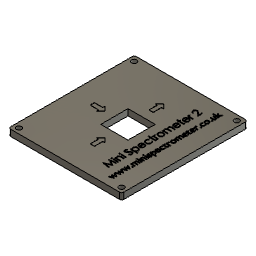
Mini Spectrometer Lid (Autodesk Fusion 360 design; units mm, degrees)
Autodesk Fusion 360 part; units mm, degrees
note: some values were not read from the file. Set by a fixed rule: which sketch regions a step uses.
(part 1 of 2)
sketch "Sketch1" plane through (0, 0, 0) normal (0, 1, 0) x (1, 0, 0)
  line L0 (-27, -30) -> (27, 30) construction
  line L1 (27, 30) -> (27, -30)
  line L2 (27, -30) -> (-27, -30)
  line L3 (-27, 30) -> (27, 30)
  line L4 (-27, -30) -> (-27, 30)
  line L5 (27, -30) -> (-27, 30) construction
  dimension "d1" = 54
  dimension "d2" = 60
  dimension "d3" = 27
  dimension "d29" = 30
  constraint horizontal L2
  constraint perpendicular L2 L4
  constraint parallel L2 L3
  constraint parallel L1 L4
  constraint coincident origin L5
  constraint coincident origin L0
  measures "d1" distance of L3.start L0.end
  measures "d2" distance of L3.start L0.start
  measures "d3" distance of origin L4
  measures "d29" distance of origin L3
extrude "Extrude1" add sketch "Sketch1" along normal blind 3
fillet "Fillet1" radius 1 4 edges at (27, 1.5, 30) (-27, 1.5, 30) (-27, 1.5, -30) (27, 1.5, -30)
sketch "Sketch3" plane through (0, 3, 0) normal (0, 1, 0) x (-1, 0, 0)
  arc A0 (-27, -29) -> (-26, -30) centre (-26, -29) ccw
  line L0 (-26, -30) -> (26, -30)
  arc A1 (26, -30) -> (27, -29) centre (26, -29) ccw
  line L1 (27, -29) -> (27, 29)
  arc A2 (27, 29) -> (26, 30) centre (26, 29) ccw
  line L2 (26, 30) -> (-26, 30)
  arc A3 (-26, 30) -> (-27, 29) centre (-26, 29) ccw
  line L3 (-27, 29) -> (-27, -29)
  circle A4 centre (24.5, -27.5) radius 1.25
  circle A5 centre (-24.5, -27.5) radius 1.25
  circle A6 centre (-24.5, 27.5) radius 1.25
  circle A7 centre (24.5, 27.5) radius 1.25
  line L4 (-6.5, -6.5) -> (-6.5, 6.5)
  line L5 (-6.5, 6.5) -> (6.5, 6.5)
  line L6 (6.5, 6.5) -> (6.5, -6.5)
  line L7 (6.5, -6.5) -> (-6.5, -6.5)
  dimension "d21" = 2.5
  dimension "d22" = 2.5
  dimension "d23" = 2.5
  dimension "d24" = 2.5
  dimension "d25" = 13
  dimension "d26" = 13
  dimension "d30" = 2.5
  dimension "d31" = 2.5
  dimension "d32" = 2.5
  dimension "d33" = 2.5
  dimension "d34" = 2.5
  dimension "d35" = 2.5
  dimension "d36" = 2.5
  dimension "d37" = 2.5
  dimension "d38" = 20.5
  dimension "d39" = 23.5
  constraint horizontal L5
  constraint perpendicular L5 L6
  constraint parallel L5 L7
  constraint parallel L4 L6
  measures "d21" diameter of A4
  measures "d22" diameter of A5
  measures "d23" diameter of A6
  measures "d24" diameter of A7
  measures "d25" distance of L4.start L6.end
  measures "d26" distance of L6.end L5.end
  measures "d30" distance of L2 A7.centre
  measures "d31" distance of L1 A7.centre
  measures "d32" distance of L2 A6.centre
  measures "d33" distance of L3 A6.centre
  measures "d34" distance of L0 A5.centre
  measures "d35" distance of L3 A5.centre
  measures "d36" distance of L0 A4.centre
  measures "d37" distance of L1 A4.centre
  measures "d38" distance of L1 L6
  measures "d39" distance of L0 L7
extrude "Extrude2" cut sketch "Sketch3" against normal blind 3 contours A4 | A5 | A6 | A7 | L4 L5 L6 L7
sketch "Sketch4" plane through (0, 3, 0) normal (0, 1, 0) x (-1, 0, 0)
  line L0 (-6.5, 6.5) -> (6.5, 6.5)
  line L1 (6.5, 6.5) -> (6.5, -6.5)
  line L2 (6.5, -6.5) -> (-6.5, -6.5)
  line L3 (-6.5, -6.5) -> (-6.5, 6.5)
  circle A0 centre (24.5, 27.5) radius 1.25
  circle A1 centre (-24.5, -27.5) radius 1.25
  circle A2 centre (24.5, -27.5) radius 1.25
  circle A3 centre (-24.5, 27.5) radius 1.25
  arc A4 (-27, -29) -> (-26, -30) centre (-26, -29) ccw
  line L4 (-26, -30) -> (26, -30)
  arc A5 (26, -30) -> (27, -29) centre (26, -29) ccw
  line L5 (27, -29) -> (27, 29)
  arc A6 (27, 29) -> (26, 30) centre (26, 29) ccw
  line L6 (26, 30) -> (-26, 30)
  arc A7 (-26, 30) -> (-27, 29) centre (-26, 29) ccw
  line L7 (-27, 29) -> (-27, -29)
  line L8 (11, 0) -> (13, -2)
  line L9 (13, -2) -> (13, -1)
  line L10 (13, -1) -> (17, -1)
  line L11 (17, -1) -> (17, 1)
  line L12 (17, 1) -> (13, 1)
  line L13 (13, 1) -> (13, 2)
  line L14 (13, 2) -> (11, 0)
  line L15 (13, -1) -> (17, -1)
  line L16 (13, -2) -> (13, -1)
  line L17 (11, 0) -> (13, -2)
  line L18 (13, 1) -> (13, 2)
  line L19 (17, 1) -> (13, 1)
  line L20 (17, -1) -> (17, 1)
  line L21 (13, 2) -> (11, 0)
  line L22 (1, 13) -> (1, 17)
  line L23 (2, 13) -> (1, 13)
  line L24 (0, 11) -> (2, 13)
  line L25 (-1, 13) -> (-2, 13)
  line L26 (-1, 17) -> (-1, 13)
  line L27 (1, 17) -> (-1, 17)
  line L28 (-2, 13) -> (0, 11)
  line L29 (1, -15) -> (1, -11)
  line L30 (2, -15) -> (1, -15)
  line L31 (0, -17) -> (2, -15)
  line L32 (-1, -15) -> (-2, -15)
  line L33 (-1, -11) -> (-1, -15)
  line L34 (1, -11) -> (-1, -11)
  line L35 (-2, -15) -> (0, -17)
  constraint perpendicular L2 L9
  constraint perpendicular L9 L10
  constraint perpendicular L10 L11
  constraint perpendicular L11 L12
  constraint perpendicular L12 L13
  constraint perpendicular L8 L14
  constraint perpendicular L15 L16
  constraint perpendicular L15 L20
  constraint perpendicular L19 L20
  constraint perpendicular L18 L19
  constraint perpendicular L17 L21
  constraint perpendicular L22 L23
  constraint perpendicular L22 L27
  constraint perpendicular L26 L27
  constraint perpendicular L25 L26
  constraint perpendicular L24 L28
  constraint perpendicular L29 L30
  constraint perpendicular L29 L34
  constraint perpendicular L33 L34
  constraint perpendicular L32 L33
  constraint perpendicular L31 L35
extrude "Extrude3" cut sketch "Sketch4" against normal blind 0.1 contours L8 L9 L10 L11 L12 L13 L14 L15 L16 L17 L18 L19 L20 L21 | L22 L23 L24 L25 L26 L27 L28 | L29 L30 L31 L32 L33 L34 L35
sketch "Sketch5" plane through (0, 3, 0) normal (0, 1, 0) x (-1, 0, 0)
  line L0 (2, -15) -> (0, -17)
  line L1 (0, -17) -> (-2, -15)
  line L2 (-2, -15) -> (-1, -15)
  line L3 (-1, -15) -> (-1, -11)
  line L4 (-1, -11) -> (1, -11)
  line L5 (1, -11) -> (1, -15)
  line L6 (1, -15) -> (2, -15)
  line L7 (2, 13) -> (0, 11)
  line L8 (0, 11) -> (-2, 13)
  line L9 (-2, 13) -> (-1, 13)
  line L10 (-1, 13) -> (-1, 17)
  line L11 (-1, 17) -> (1, 17)
  line L12 (1, 17) -> (1, 13)
  line L13 (1, 13) -> (2, 13)
  line L14 (13, -2) -> (11, 0)
  line L15 (11, 0) -> (13, 2)
  line L16 (13, 2) -> (13, 1)
  line L17 (13, 1) -> (17, 1)
  line L18 (17, 1) -> (17, -1)
  line L19 (17, -1) -> (13, -1)
  line L20 (13, -1) -> (13, -2)
  line L21 (-6.5, 6.5) -> (6.5, 6.5)
  line L22 (6.5, 6.5) -> (6.5, -6.5)
  line L23 (6.5, -6.5) -> (-6.5, -6.5)
  line L24 (-6.5, -6.5) -> (-6.5, 6.5)
  circle A0 centre (24.5, 27.5) radius 1.25
  circle A1 centre (-24.5, -27.5) radius 1.25
  circle A2 centre (24.5, -27.5) radius 1.25
  circle A3 centre (-24.5, 27.5) radius 1.25
  arc A4 (-27, -29) -> (-26, -30) centre (-26, -29) ccw
  line L25 (-26, -30) -> (26, -30)
  arc A5 (26, -30) -> (27, -29) centre (26, -29) ccw
  line L26 (27, -29) -> (27, 29)
  arc A6 (27, 29) -> (26, 30) centre (26, 29) ccw
  line L27 (26, 30) -> (-26, 30)
  arc A7 (-26, 30) -> (-27, 29) centre (-26, 29) ccw
  line L28 (-27, 29) -> (-27, -29)
  line L29 (-13.2189, 22.3541) -> (-9.8548, 21.8762)
  line L30 (-9.8548, 21.8762) -> (-9.8548, 21.8246)
  line L31 (-9.8548, 21.8246) -> (-12.6145, 20.4565)
  line L32 (-12.6145, 20.4565) -> (-9.8548, 19.0977)
  line L33 (-9.8548, 19.0977) -> (-9.8548, 19.0462)
  line L34 (-9.8548, 19.0462) -> (-13.2189, 18.5636)
  line L35 (-13.2189, 18.5636) -> (-13.2189, 18.8963)
  line L36 (-13.2189, 18.8963) -> (-10.8106, 19.2242)
  line L37 (-10.8106, 19.2242) -> (-13.2189, 20.4143)
  line L38 (-13.2189, 20.4143) -> (-13.2189, 20.4987)
  line L39 (-13.2189, 20.4987) -> (-10.7918, 21.7028)
  line L40 (-10.7918, 21.7028) -> (-13.2189, 22.0308)
  line L41 (-13.2189, 22.0308) -> (-13.2189, 22.3541)
  spline S0 degree 2 poles (-10.0375, 18.0997) (-9.9297, 18.0997) (-9.8501, 18.0248) knots 0 0 0 1 1 1
  spline S1 degree 2 poles (-9.8501, 18.0248) (-9.7704, 17.9451) (-9.7704, 17.8373) knots 0 0 0 1 1 1
  spline S2 degree 2 poles (-9.7704, 17.8373) (-9.7704, 17.7249) (-9.8501, 17.6499) knots 0 0 0 1 1 1
  spline S3 degree 2 poles (-9.8501, 17.6499) (-9.925, 17.5703) (-10.0375, 17.5703) knots 0 0 0 1 1 1
  spline S4 degree 2 poles (-10.0375, 17.5703) (-10.1452, 17.5703) (-10.2249, 17.6499) knots 0 0 0 1 1 1
  spline S5 degree 2 poles (-10.2249, 17.6499) (-10.2999, 17.7249) (-10.2999, 17.8373) knots 0 0 0 1 1 1
  spline S6 degree 2 poles (-10.2999, 17.8373) (-10.2999, 17.9451) (-10.2202, 18.0248) knots 0 0 0 1 1 1
  spline S7 degree 2 poles (-10.2202, 18.0248) (-10.1406, 18.0997) (-10.0375, 18.0997) knots 0 0 0 1 1 1
  line L42 (-10.7309, 17.9967) -> (-10.7309, 17.6734)
  line L43 (-10.7309, 17.6734) -> (-13.2189, 17.6734)
  line L44 (-13.2189, 17.6734) -> (-13.2189, 17.9967)
  line L45 (-13.2189, 17.9967) -> (-10.7309, 17.9967)
  line L46 (-10.7309, 17.0127) -> (-10.7309, 16.6894)
  line L47 (-10.7309, 16.6894) -> (-11.176, 16.6894)
  spline S8 degree 2 poles (-11.176, 16.6894) (-10.6653, 16.3052) (-10.6653, 15.757) knots 0 0 0 1 1 1
  spline S9 degree 2 poles (-10.6653, 15.757) (-10.6653, 15.4759) (-10.8199, 15.251) knots 0 0 0 1 1 1
  spline S10 degree 2 poles (-10.8199, 15.251) (-10.9699, 15.0261) (-11.2182, 14.9324) knots 0 0 0 1 1 1
  spline S11 degree 2 poles (-11.2182, 14.9324) (-11.4618, 14.8387) (-11.9398, 14.8387) knots 0 0 0 1 1 1
  line L48 (-11.9398, 14.8387) -> (-13.2189, 14.8387)
  line L49 (-13.2189, 14.8387) -> (-13.2189, 15.1573)
  line L50 (-13.2189, 15.1573) -> (-12.0335, 15.1573)
  spline S12 degree 2 poles (-12.0335, 15.1573) (-11.5977, 15.1573) (-11.4431, 15.1995) knots 0 0 0 1 1 1
  spline S13 degree 2 poles (-11.4431, 15.1995) (-11.2885, 15.2369) (-11.1807, 15.3213) knots 0 0 0 1 1 1
  spline S14 degree 2 poles (-11.1807, 15.3213) (-11.073, 15.4009) (-11.0167, 15.5274) knots 0 0 0 1 1 1
  spline S15 degree 2 poles (-11.0167, 15.5274) (-10.9605, 15.6539) (-10.9605, 15.8367) knots 0 0 0 1 1 1
  spline S16 degree 2 poles (-10.9605, 15.8367) (-10.9605, 16.0147) (-11.0495, 16.1881) knots 0 0 0 1 1 1
  spline S17 degree 2 poles (-11.0495, 16.1881) (-11.1386, 16.3614) (-11.2979, 16.4833) knots 0 0 0 1 1 1
  spline S18 degree 2 poles (-11.2979, 16.4833) (-11.4572, 16.6051) (-11.6258, 16.6473) knots 0 0 0 1 1 1
  spline S19 degree 2 poles (-11.6258, 16.6473) (-11.7945, 16.6894) (-12.3052, 16.6894) knots 0 0 0 1 1 1
  line L51 (-12.3052, 16.6894) -> (-13.2189, 16.6894)
  line L52 (-13.2189, 16.6894) -> (-13.2189, 17.0127)
  line L53 (-13.2189, 17.0127) -> (-10.7309, 17.0127)
  spline S20 degree 2 poles (-10.0375, 14.3046) (-9.9297, 14.3046) (-9.8501, 14.2296) knots 0 0 0 1 1 1
  spline S21 degree 2 poles (-9.8501, 14.2296) (-9.7704, 14.1499) (-9.7704, 14.0422) knots 0 0 0 1 1 1
  spline S22 degree 2 poles (-9.7704, 14.0422) (-9.7704, 13.9297) (-9.8501, 13.8548) knots 0 0 0 1 1 1
  spline S23 degree 2 poles (-9.8501, 13.8548) (-9.925, 13.7751) (-10.0375, 13.7751) knots 0 0 0 1 1 1
  spline S24 degree 2 poles (-10.0375, 13.7751) (-10.1452, 13.7751) (-10.2249, 13.8548) knots 0 0 0 1 1 1
  spline S25 degree 2 poles (-10.2249, 13.8548) (-10.2999, 13.9297) (-10.2999, 14.0422) knots 0 0 0 1 1 1
  spline S26 degree 2 poles (-10.2999, 14.0422) (-10.2999, 14.1499) (-10.2202, 14.2296) knots 0 0 0 1 1 1
  spline S27 degree 2 poles (-10.2202, 14.2296) (-10.1406, 14.3046) (-10.0375, 14.3046) knots 0 0 0 1 1 1
  line L54 (-10.7309, 14.2015) -> (-10.7309, 13.8782)
  line L55 (-10.7309, 13.8782) -> (-13.2189, 13.8782)
  line L56 (-13.2189, 13.8782) -> (-13.2189, 14.2015)
  line L57 (-13.2189, 14.2015) -> (-10.7309, 14.2015)
  line L58 (-12.591, 12.3414) -> (-12.4224, 12.0556)
  spline S28 degree 2 poles (-12.4224, 12.0556) (-12.9752, 11.7557) (-12.9752, 11.3574) knots 0 0 0 1 1 1
  spline S29 degree 2 poles (-12.9752, 11.3574) (-12.9752, 11.0997) (-12.8112, 10.917) knots 0 0 0 1 1 1
  spline S30 degree 2 poles (-12.8112, 10.917) (-12.6473, 10.7343) (-12.4036, 10.7343) knots 0 0 0 1 1 1
  spline S31 degree 2 poles (-12.4036, 10.7343) (-12.2115, 10.7343) (-12.0147, 10.8889) knots 0 0 0 1 1 1
  spline S32 degree 2 poles (-12.0147, 10.8889) (-11.8179, 11.0435) (-11.5509, 11.4043) knots 0 0 0 1 1 1
  spline S33 degree 2 poles (-11.5509, 11.4043) (-11.2791, 11.7604) (-11.1479, 11.8869) knots 0 0 0 1 1 1
  spline S34 degree 2 poles (-11.1479, 11.8869) (-11.012, 12.0087) (-10.8621, 12.0696) knots 0 0 0 1 1 1
  spline S35 degree 2 poles (-10.8621, 12.0696) (-10.7075, 12.1258) (-10.5529, 12.1258) knots 0 0 0 1 1 1
  spline S36 degree 2 poles (-10.5529, 12.1258) (-10.2249, 12.1258) (-10, 11.8963) knots 0 0 0 1 1 1
  spline S37 degree 2 poles (-10, 11.8963) (-9.7704, 11.662) (-9.7704, 11.3106) knots 0 0 0 1 1 1
  spline S38 degree 2 poles (-9.7704, 11.3106) (-9.7704, 11.0341) (-9.911, 10.828) knots 0 0 0 1 1 1
  spline S39 degree 2 poles (-9.911, 10.828) (-10.0469, 10.6218) (-10.3186, 10.4297) knots 0 0 0 1 1 1
  line L59 (-10.3186, 10.4297) -> (-10.5295, 10.7015)
  spline S40 degree 2 poles (-10.5295, 10.7015) (-10.3514, 10.8327) (-10.2343, 10.9732) knots 0 0 0 1 1 1
  spline S41 degree 2 poles (-10.2343, 10.9732) (-10.1171, 11.1138) (-10.1171, 11.3199) knots 0 0 0 1 1 1
  spline S42 degree 2 poles (-10.1171, 11.3199) (-10.1171, 11.5214) (-10.239, 11.6526) knots 0 0 0 1 1 1
  spline S43 degree 2 poles (-10.239, 11.6526) (-10.3608, 11.7791) (-10.5482, 11.7791) knots 0 0 0 1 1 1
  spline S44 degree 2 poles (-10.5482, 11.7791) (-10.7356, 11.7791) (-10.8762, 11.6667) knots 0 0 0 1 1 1
  spline S45 degree 2 poles (-10.8762, 11.6667) (-11.012, 11.5495) (-11.3119, 11.1466) knots 0 0 0 1 1 1
  spline S46 degree 2 poles (-11.3119, 11.1466) (-11.6118, 10.739) (-11.8648, 10.5562) knots 0 0 0 1 1 1
  spline S47 degree 2 poles (-11.8648, 10.5562) (-12.1178, 10.3688) (-12.3989, 10.3688) knots 0 0 0 1 1 1
  spline S48 degree 2 poles (-12.3989, 10.3688) (-12.7644, 10.3688) (-13.0361, 10.6546) knots 0 0 0 1 1 1
  spline S49 degree 2 poles (-13.0361, 10.6546) (-13.3032, 10.9357) (-13.3032, 11.3106) knots 0 0 0 1 1 1
  spline S50 degree 2 poles (-13.3032, 11.3106) (-13.3032, 11.9712) (-12.591, 12.3414) knots 0 0 0 1 1 1
  line L60 (-10.7309, 9.7082) -> (-10.7309, 9.3896)
  line L61 (-10.7309, 9.3896) -> (-11.1854, 9.3896)
  spline S51 degree 2 poles (-11.1854, 9.3896) (-10.6653, 9.01) (-10.6653, 8.4009) knots 0 0 0 1 1 1
  spline S52 degree 2 poles (-10.6653, 8.4009) (-10.6653, 7.8762) (-11.0542, 7.4967) knots 0 0 0 1 1 1
  spline S53 degree 2 poles (-11.0542, 7.4967) (-11.4384, 7.1171) (-11.9819, 7.1171) knots 0 0 0 1 1 1
  spline S54 degree 2 poles (-11.9819, 7.1171) (-12.5254, 7.1171) (-12.9143, 7.492) knots 0 0 0 1 1 1
  spline S55 degree 2 poles (-12.9143, 7.492) (-13.3032, 7.8668) (-13.3032, 8.3916) knots 0 0 0 1 1 1
  spline S56 degree 2 poles (-13.3032, 8.3916) (-13.3032, 8.9632) (-12.7925, 9.3896) knots 0 0 0 1 1 1
  line L62 (-12.7925, 9.3896) -> (-14.1278, 9.3896)
  line L63 (-14.1278, 9.3896) -> (-14.1278, 9.7082)
  line L64 (-14.1278, 9.7082) -> (-10.7309, 9.7082)
  spline S57 degree 2 poles (-11.9866, 7.4357) (-11.5696, 7.4357) (-11.2744, 7.7262) knots 0 0 0 1 1 1
  spline S58 degree 2 poles (-11.2744, 7.7262) (-10.9746, 8.012) (-10.9746, 8.429) knots 0 0 0 1 1 1
  spline S59 degree 2 poles (-10.9746, 8.429) (-10.9746, 8.846) (-11.2697, 9.1319) knots 0 0 0 1 1 1
  spline S60 degree 2 poles (-11.2697, 9.1319) (-11.5602, 9.413) (-11.9913, 9.413) knots 0 0 0 1 1 1
  spline S61 degree 2 poles (-11.9913, 9.413) (-12.4224, 9.413) (-12.7175, 9.1225) knots 0 0 0 1 1 1
  spline S62 degree 2 poles (-12.7175, 9.1225) (-13.008, 8.832) (-13.008, 8.429) knots 0 0 0 1 1 1
  spline S63 degree 2 poles (-13.008, 8.429) (-13.008, 8.0214) (-12.7129, 7.7309) knots 0 0 0 1 1 1
  spline S64 degree 2 poles (-12.7129, 7.7309) (-12.413, 7.4357) (-11.9866, 7.4357) knots 0 0 0 1 1 1
  line L65 (-12.413, 4.423) -> (-12.5535, 4.1513)
  spline S65 degree 2 poles (-12.5535, 4.1513) (-13.3032, 4.5542) (-13.3032, 5.3414) knots 0 0 0 1 1 1
  spline S66 degree 2 poles (-13.3032, 5.3414) (-13.3032, 5.9036) (-12.919, 6.2691) knots 0 0 0 1 1 1
  spline S67 degree 2 poles (-12.919, 6.2691) (-12.5301, 6.6345) (-11.9866, 6.6345) knots 0 0 0 1 1 1
  spline S68 degree 2 poles (-11.9866, 6.6345) (-11.4431, 6.6345) (-11.0542, 6.2691) knots 0 0 0 1 1 1
  spline S69 degree 2 poles (-11.0542, 6.2691) (-10.6653, 5.8989) (-10.6653, 5.3601) knots 0 0 0 1 1 1
  spline S70 degree 2 poles (-10.6653, 5.3601) (-10.6653, 4.8166) (-11.0261, 4.4511) knots 0 0 0 1 1 1
  spline S71 degree 2 poles (-11.0261, 4.4511) (-11.3869, 4.081) (-12.01, 4.0669) knots 0 0 0 1 1 1
  line L66 (-12.01, 4.0669) -> (-12.01, 6.3066)
  spline S72 degree 2 poles (-12.01, 6.3066) (-12.4598, 6.2925) (-12.7363, 6.0254) knots 0 0 0 1 1 1
  spline S73 degree 2 poles (-12.7363, 6.0254) (-13.008, 5.7537) (-13.008, 5.3695) knots 0 0 0 1 1 1
  spline S74 degree 2 poles (-13.008, 5.3695) (-13.008, 4.7369) (-12.413, 4.423) knots 0 0 0 1 1 1
  spline S75 degree 2 poles (-11.7336, 4.423) (-11.3775, 4.4886) (-11.176, 4.751) knots 0 0 0 1 1 1
  spline S76 degree 2 poles (-11.176, 4.751) (-10.9746, 5.0134) (-10.9746, 5.3554) knots 0 0 0 1 1 1
  spline S77 degree 2 poles (-10.9746, 5.3554) (-10.9746, 6.0582) (-11.7336, 6.2738) knots 0 0 0 1 1 1
  line L67 (-11.7336, 6.2738) -> (-11.7336, 4.423)
  line L68 (-11.2463, 1.0402) -> (-11.4056, 1.2932)
  spline S78 degree 2 poles (-11.4056, 1.2932) (-10.9699, 1.6212) (-10.9699, 2.1928) knots 0 0 0 1 1 1
  spline S79 degree 2 poles (-10.9699, 2.1928) (-10.9699, 2.6426) (-11.2604, 2.9471) knots 0 0 0 1 1 1
  spline S80 degree 2 poles (-11.2604, 2.9471) (-11.5462, 3.2517) (-11.9726, 3.2517) knots 0 0 0 1 1 1
  spline S81 degree 2 poles (-11.9726, 3.2517) (-12.3989, 3.2517) (-12.7035, 2.9518) knots 0 0 0 1 1 1
  spline S82 degree 2 poles (-12.7035, 2.9518) (-13.008, 2.6519) (-13.008, 2.1928) knots 0 0 0 1 1 1
  spline S83 degree 2 poles (-13.008, 2.1928) (-13.008, 1.6446) (-12.5723, 1.2932) knots 0 0 0 1 1 1
  line L69 (-12.5723, 1.2932) -> (-12.741, 1.0402)
  spline S84 degree 2 poles (-12.741, 1.0402) (-13.0127, 1.2276) (-13.158, 1.5462) knots 0 0 0 1 1 1
  spline S85 degree 2 poles (-13.158, 1.5462) (-13.3032, 1.8601) (-13.3032, 2.2256) knots 0 0 0 1 1 1
  spline S86 degree 2 poles (-13.3032, 2.2256) (-13.3032, 2.8019) (-12.9237, 3.1908) knots 0 0 0 1 1 1
  spline S87 degree 2 poles (-12.9237, 3.1908) (-12.5442, 3.575) (-11.996, 3.575) knots 0 0 0 1 1 1
  spline S88 degree 2 poles (-11.996, 3.575) (-11.4478, 3.575) (-11.0589, 3.1861) knots 0 0 0 1 1 1
  spline S89 degree 2 poles (-11.0589, 3.1861) (-10.6653, 2.7925) (-10.6653, 2.1787) knots 0 0 0 1 1 1
  spline S90 degree 2 poles (-10.6653, 2.1787) (-10.6653, 1.8179) (-10.8199, 1.5134) knots 0 0 0 1 1 1
  spline S91 degree 2 poles (-10.8199, 1.5134) (-10.9746, 1.2041) (-11.2463, 1.0402) knots 0 0 0 1 1 1
  spline S92 degree 2 poles (-12.8253, -0.164) (-12.9518, -0.164) (-12.9752, -0.1968) knots 0 0 0 1 1 1
  spline S93 degree 2 poles (-12.9752, -0.1968) (-12.9987, -0.2296) (-12.9987, -0.3655) knots 0 0 0 1 1 1
  line L70 (-12.9987, -0.3655) -> (-12.9987, -0.5576)
  line L71 (-12.9987, -0.5576) -> (-13.2704, -0.5576)
  spline S94 degree 2 poles (-13.2704, -0.5576) (-13.3032, -0.3608) (-13.3032, -0.2483) knots 0 0 0 1 1 1
  spline S95 degree 2 poles (-13.3032, -0.2483) (-13.3032, -0.0375) (-13.2001, 0.0609) knots 0 0 0 1 1 1
  spline S96 degree 2 poles (-13.2001, 0.0609) (-13.0971, 0.1593) (-12.8768, 0.1593) knots 0 0 0 1 1 1
  line L72 (-12.8768, 0.1593) -> (-11.0027, 0.1593)
  line L73 (-11.0027, 0.1593) -> (-11.0027, 0.5997)
  line L74 (-11.0027, 0.5997) -> (-10.7309, 0.5997)
  line L75 (-10.7309, 0.5997) -> (-10.7309, 0.1593)
  line L76 (-10.7309, 0.1593) -> (-9.7704, 0.1593)
  line L77 (-9.7704, 0.1593) -> (-9.7704, -0.164)
  line L78 (-9.7704, -0.164) -> (-10.7309, -0.164)
  line L79 (-10.7309, -0.164) -> (-10.7309, -0.67)
  line L80 (-10.7309, -0.67) -> (-11.0027, -0.67)
  line L81 (-11.0027, -0.67) -> (-11.0027, -0.164)
  line L82 (-11.0027, -0.164) -> (-12.8253, -0.164)
  line L83 (-10.7309, -1.0261) -> (-10.7309, -1.3541)
  line L84 (-10.7309, -1.3541) -> (-11.0917, -1.3541)
  spline S97 degree 2 poles (-11.0917, -1.3541) (-10.8715, -1.4853) (-10.7684, -1.6071) knots 0 0 0 1 1 1
  spline S98 degree 2 poles (-10.7684, -1.6071) (-10.6653, -1.7336) (-10.6653, -1.8835) knots 0 0 0 1 1 1
  spline S99 degree 2 poles (-10.6653, -1.8835) (-10.6653, -2.0382) (-10.7497, -2.1928) knots 0 0 0 1 1 1
  line L85 (-10.7497, -2.1928) -> (-11.0214, -2.0241)
  spline S100 degree 2 poles (-11.0214, -2.0241) (-10.9793, -1.9538) (-10.9793, -1.8789) knots 0 0 0 1 1 1
  spline S101 degree 2 poles (-10.9793, -1.8789) (-10.9793, -1.7336) (-11.1292, -1.6024) knots 0 0 0 1 1 1
  spline S102 degree 2 poles (-11.1292, -1.6024) (-11.2791, -1.4759) (-11.5181, -1.415) knots 0 0 0 1 1 1
  spline S103 degree 2 poles (-11.5181, -1.415) (-11.7523, -1.3541) (-12.3755, -1.3541) knots 0 0 0 1 1 1
  line L86 (-12.3755, -1.3541) -> (-13.2189, -1.3541)
  line L87 (-13.2189, -1.3541) -> (-13.2189, -1.0261)
  line L88 (-13.2189, -1.0261) -> (-10.7309, -1.0261)
  spline S104 degree 2 poles (-11.9913, -2.4411) (-11.4431, -2.4411) (-11.0542, -2.8159) knots 0 0 0 1 1 1
  spline S105 degree 2 poles (-11.0542, -2.8159) (-10.6653, -3.1955) (-10.6653, -3.7343) knots 0 0 0 1 1 1
  spline S106 degree 2 poles (-10.6653, -3.7343) (-10.6653, -4.2778) (-11.0542, -4.6526) knots 0 0 0 1 1 1
  spline S107 degree 2 poles (-11.0542, -4.6526) (-11.4431, -5.0321) (-11.9866, -5.0321) knots 0 0 0 1 1 1
  spline S108 degree 2 poles (-11.9866, -5.0321) (-12.5301, -5.0321) (-12.919, -4.6573) knots 0 0 0 1 1 1
  spline S109 degree 2 poles (-12.919, -4.6573) (-13.3032, -4.2872) (-13.3032, -3.739) knots 0 0 0 1 1 1
  spline S110 degree 2 poles (-13.3032, -3.739) (-13.3032, -3.1908) (-12.919, -2.8159) knots 0 0 0 1 1 1
  spline S111 degree 2 poles (-12.919, -2.8159) (-12.5301, -2.4411) (-11.9913, -2.4411) knots 0 0 0 1 1 1
  spline S112 degree 2 poles (-11.996, -4.7088) (-11.5837, -4.7088) (-11.2838, -4.4183) knots 0 0 0 1 1 1
  spline S113 degree 2 poles (-11.2838, -4.4183) (-10.9793, -4.1325) (-10.9793, -3.7343) knots 0 0 0 1 1 1
  spline S114 degree 2 poles (-10.9793, -3.7343) (-10.9793, -3.3407) (-11.2838, -3.0549) knots 0 0 0 1 1 1
  spline S115 degree 2 poles (-11.2838, -3.0549) (-11.5837, -2.7691) (-12.0007, -2.7691) knots 0 0 0 1 1 1
  spline S116 degree 2 poles (-12.0007, -2.7691) (-12.4177, -2.7691) (-12.7082, -3.0455) knots 0 0 0 1 1 1
  spline S117 degree 2 poles (-12.7082, -3.0455) (-12.9987, -3.322) (-12.9987, -3.7296) knots 0 0 0 1 1 1
  spline S118 degree 2 poles (-12.9987, -3.7296) (-12.9987, -4.1419) (-12.7082, -4.423) knots 0 0 0 1 1 1
  spline S119 degree 2 poles (-12.7082, -4.423) (-12.413, -4.7088) (-11.996, -4.7088) knots 0 0 0 1 1 1
  line L89 (-10.7309, -5.6272) -> (-10.7309, -5.9458)
  line L90 (-10.7309, -5.9458) -> (-11.162, -5.9458)
  spline S120 degree 2 poles (-11.162, -5.9458) (-10.6653, -6.2785) (-10.6653, -6.7985) knots 0 0 0 1 1 1
  spline S121 degree 2 poles (-10.6653, -6.7985) (-10.6653, -7.075) (-10.8246, -7.2905) knots 0 0 0 1 1 1
  spline S122 degree 2 poles (-10.8246, -7.2905) (-10.9793, -7.5107) (-11.2651, -7.5857) knots 0 0 0 1 1 1
  spline S123 degree 2 poles (-11.2651, -7.5857) (-10.9746, -7.7403) (-10.8199, -7.9793) knots 0 0 0 1 1 1
  spline S124 degree 2 poles (-10.8199, -7.9793) (-10.6653, -8.2182) (-10.6653, -8.5274) knots 0 0 0 1 1 1
  spline S125 degree 2 poles (-10.6653, -8.5274) (-10.6653, -8.8414) (-10.909, -9.0944) knots 0 0 0 1 1 1
  spline S126 degree 2 poles (-10.909, -9.0944) (-11.1479, -9.3474) (-11.8601, -9.3474) knots 0 0 0 1 1 1
  line L91 (-11.8601, -9.3474) -> (-13.2189, -9.3474)
  line L92 (-13.2189, -9.3474) -> (-13.2189, -9.0194)
  line L93 (-13.2189, -9.0194) -> (-11.8601, -9.0194)
  spline S127 degree 2 poles (-11.8601, -9.0194) (-11.5181, -9.0194) (-11.3588, -8.9772) knots 0 0 0 1 1 1
  spline S128 degree 2 poles (-11.3588, -8.9772) (-11.1948, -8.9351) (-11.087, -8.7945) knots 0 0 0 1 1 1
  spline S129 degree 2 poles (-11.087, -8.7945) (-10.9746, -8.654) (-10.9746, -8.4197) knots 0 0 0 1 1 1
  spline S130 degree 2 poles (-10.9746, -8.4197) (-10.9746, -8.1901) (-11.1292, -7.9886) knots 0 0 0 1 1 1
  spline S131 degree 2 poles (-11.1292, -7.9886) (-11.2838, -7.7872) (-11.5228, -7.7122) knots 0 0 0 1 1 1
  spline S132 degree 2 poles (-11.5228, -7.7122) (-11.7617, -7.6372) (-12.2443, -7.6372) knots 0 0 0 1 1 1
  line L94 (-12.2443, -7.6372) -> (-13.2189, -7.6372)
  line L95 (-13.2189, -7.6372) -> (-13.2189, -7.3233)
  line L96 (-13.2189, -7.3233) -> (-11.9444, -7.3233)
  spline S133 degree 2 poles (-11.9444, -7.3233) (-11.5462, -7.3233) (-11.3775, -7.2811) knots 0 0 0 1 1 1
  spline S134 degree 2 poles (-11.3775, -7.2811) (-11.2041, -7.239) (-11.0917, -7.0937) knots 0 0 0 1 1 1
  spline S135 degree 2 poles (-11.0917, -7.0937) (-10.9746, -6.9485) (-10.9746, -6.7376) knots 0 0 0 1 1 1
  spline S136 degree 2 poles (-10.9746, -6.7376) (-10.9746, -6.5268) (-11.1011, -6.3394) knots 0 0 0 1 1 1
  spline S137 degree 2 poles (-11.1011, -6.3394) (-11.2229, -6.1566) (-11.4384, -6.0489) knots 0 0 0 1 1 1
  spline S138 degree 2 poles (-11.4384, -6.0489) (-11.6539, -5.9458) (-12.1647, -5.9458) knots 0 0 0 1 1 1
  line L97 (-12.1647, -5.9458) -> (-13.2189, -5.9458)
  line L98 (-13.2189, -5.9458) -> (-13.2189, -5.6272)
  line L99 (-13.2189, -5.6272) -> (-10.7309, -5.6272)
  line L100 (-12.413, -12.1165) -> (-12.5535, -12.3882)
  spline S139 degree 2 poles (-12.5535, -12.3882) (-13.3032, -11.9853) (-13.3032, -11.1981) knots 0 0 0 1 1 1
  spline S140 degree 2 poles (-13.3032, -11.1981) (-13.3032, -10.6359) (-12.919, -10.2704) knots 0 0 0 1 1 1
  spline S141 degree 2 poles (-12.919, -10.2704) (-12.5301, -9.905) (-11.9866, -9.905) knots 0 0 0 1 1 1
  spline S142 degree 2 poles (-11.9866, -9.905) (-11.4431, -9.905) (-11.0542, -10.2704) knots 0 0 0 1 1 1
  spline S143 degree 2 poles (-11.0542, -10.2704) (-10.6653, -10.6406) (-10.6653, -11.1794) knots 0 0 0 1 1 1
  spline S144 degree 2 poles (-10.6653, -11.1794) (-10.6653, -11.7229) (-11.0261, -12.0884) knots 0 0 0 1 1 1
  spline S145 degree 2 poles (-11.0261, -12.0884) (-11.3869, -12.4585) (-12.01, -12.4726) knots 0 0 0 1 1 1
  line L101 (-12.01, -12.4726) -> (-12.01, -10.2329)
  spline S146 degree 2 poles (-12.01, -10.2329) (-12.4598, -10.247) (-12.7363, -10.5141) knots 0 0 0 1 1 1
  spline S147 degree 2 poles (-12.7363, -10.5141) (-13.008, -10.7858) (-13.008, -11.17) knots 0 0 0 1 1 1
  spline S148 degree 2 poles (-13.008, -11.17) (-13.008, -11.8025) (-12.413, -12.1165) knots 0 0 0 1 1 1
  spline S149 degree 2 poles (-11.7336, -12.1165) (-11.3775, -12.0509) (-11.176, -11.7885) knots 0 0 0 1 1 1
  spline S150 degree 2 poles (-11.176, -11.7885) (-10.9746, -11.5261) (-10.9746, -11.1841) knots 0 0 0 1 1 1
  spline S151 degree 2 poles (-10.9746, -11.1841) (-10.9746, -10.4813) (-11.7336, -10.2657) knots 0 0 0 1 1 1
  line L102 (-11.7336, -10.2657) -> (-11.7336, -12.1165)
  spline S152 degree 2 poles (-12.8253, -13.672) (-12.9518, -13.672) (-12.9752, -13.7048) knots 0 0 0 1 1 1
  spline S153 degree 2 poles (-12.9752, -13.7048) (-12.9987, -13.7376) (-12.9987, -13.8735) knots 0 0 0 1 1 1
  line L103 (-12.9987, -13.8735) -> (-12.9987, -14.0656)
  line L104 (-12.9987, -14.0656) -> (-13.2704, -14.0656)
  spline S154 degree 2 poles (-13.2704, -14.0656) (-13.3032, -13.8688) (-13.3032, -13.7564) knots 0 0 0 1 1 1
  spline S155 degree 2 poles (-13.3032, -13.7564) (-13.3032, -13.5455) (-13.2001, -13.4471) knots 0 0 0 1 1 1
  spline S156 degree 2 poles (-13.2001, -13.4471) (-13.0971, -13.3487) (-12.8768, -13.3487) knots 0 0 0 1 1 1
  line L105 (-12.8768, -13.3487) -> (-11.0027, -13.3487)
  line L106 (-11.0027, -13.3487) -> (-11.0027, -12.9083)
  line L107 (-11.0027, -12.9083) -> (-10.7309, -12.9083)
  line L108 (-10.7309, -12.9083) -> (-10.7309, -13.3487)
  line L109 (-10.7309, -13.3487) -> (-9.7704, -13.3487)
  line L110 (-9.7704, -13.3487) -> (-9.7704, -13.672)
  line L111 (-9.7704, -13.672) -> (-10.7309, -13.672)
  line L112 (-10.7309, -13.672) -> (-10.7309, -14.178)
  line L113 (-10.7309, -14.178) -> (-11.0027, -14.178)
  line L114 (-11.0027, -14.178) -> (-11.0027, -13.672)
  line L115 (-11.0027, -13.672) -> (-12.8253, -13.672)
  line L116 (-12.413, -16.7503) -> (-12.5535, -17.0221)
  spline S157 degree 2 poles (-12.5535, -17.0221) (-13.3032, -16.6191) (-13.3032, -15.832) knots 0 0 0 1 1 1
  spline S158 degree 2 poles (-13.3032, -15.832) (-13.3032, -15.2697) (-12.919, -14.9043) knots 0 0 0 1 1 1
  spline S159 degree 2 poles (-12.919, -14.9043) (-12.5301, -14.5388) (-11.9866, -14.5388) knots 0 0 0 1 1 1
  spline S160 degree 2 poles (-11.9866, -14.5388) (-11.4431, -14.5388) (-11.0542, -14.9043) knots 0 0 0 1 1 1
  spline S161 degree 2 poles (-11.0542, -14.9043) (-10.6653, -15.2744) (-10.6653, -15.8133) knots 0 0 0 1 1 1
  spline S162 degree 2 poles (-10.6653, -15.8133) (-10.6653, -16.3568) (-11.0261, -16.7222) knots 0 0 0 1 1 1
  spline S163 degree 2 poles (-11.0261, -16.7222) (-11.3869, -17.0924) (-12.01, -17.1064) knots 0 0 0 1 1 1
  line L117 (-12.01, -17.1064) -> (-12.01, -14.8668)
  spline S164 degree 2 poles (-12.01, -14.8668) (-12.4598, -14.8809) (-12.7363, -15.1479) knots 0 0 0 1 1 1
  spline S165 degree 2 poles (-12.7363, -15.1479) (-13.008, -15.4197) (-13.008, -15.8039) knots 0 0 0 1 1 1
  spline S166 degree 2 poles (-13.008, -15.8039) (-13.008, -16.4364) (-12.413, -16.7503) knots 0 0 0 1 1 1
  spline S167 degree 2 poles (-11.7336, -16.7503) (-11.3775, -16.6847) (-11.176, -16.4224) knots 0 0 0 1 1 1
  spline S168 degree 2 poles (-11.176, -16.4224) (-10.9746, -16.16) (-10.9746, -15.8179) knots 0 0 0 1 1 1
  spline S169 degree 2 poles (-10.9746, -15.8179) (-10.9746, -15.1151) (-11.7336, -14.8996) knots 0 0 0 1 1 1
  line L118 (-11.7336, -14.8996) -> (-11.7336, -16.7503)
  line L119 (-10.7309, -17.5797) -> (-10.7309, -17.9076)
  line L120 (-10.7309, -17.9076) -> (-11.0917, -17.9076)
  spline S170 degree 2 poles (-11.0917, -17.9076) (-10.8715, -18.0388) (-10.7684, -18.1606) knots 0 0 0 1 1 1
  spline S171 degree 2 poles (-10.7684, -18.1606) (-10.6653, -18.2871) (-10.6653, -18.4371) knots 0 0 0 1 1 1
  spline S172 degree 2 poles (-10.6653, -18.4371) (-10.6653, -18.5917) (-10.7497, -18.7463) knots 0 0 0 1 1 1
  line L121 (-10.7497, -18.7463) -> (-11.0214, -18.5776)
  spline S173 degree 2 poles (-11.0214, -18.5776) (-10.9793, -18.5074) (-10.9793, -18.4324) knots 0 0 0 1 1 1
  spline S174 degree 2 poles (-10.9793, -18.4324) (-10.9793, -18.2871) (-11.1292, -18.156) knots 0 0 0 1 1 1
  spline S175 degree 2 poles (-11.1292, -18.156) (-11.2791, -18.0295) (-11.5181, -17.9685) knots 0 0 0 1 1 1
  spline S176 degree 2 poles (-11.5181, -17.9685) (-11.7523, -17.9076) (-12.3755, -17.9076) knots 0 0 0 1 1 1
  line L122 (-12.3755, -17.9076) -> (-13.2189, -17.9076)
  line L123 (-13.2189, -17.9076) -> (-13.2189, -17.5797)
  line L124 (-13.2189, -17.5797) -> (-10.7309, -17.5797)
  line L125 (-10.909, -20.4706) -> (-10.909, -20.1473)
  spline S177 degree 2 poles (-10.909, -20.1473) (-10.3936, -20.1707) (-10.0843, -20.4893) knots 0 0 0 1 1 1
  spline S178 degree 2 poles (-10.0843, -20.4893) (-9.7704, -20.8079) (-9.7704, -21.2577) knots 0 0 0 1 1 1
  spline S179 degree 2 poles (-9.7704, -21.2577) (-9.7704, -21.7122) (-10.0656, -22.0074) knots 0 0 0 1 1 1
  spline S180 degree 2 poles (-10.0656, -22.0074) (-10.3561, -22.3072) (-10.7778, -22.3072) knots 0 0 0 1 1 1
  spline S181 degree 2 poles (-10.7778, -22.3072) (-11.0917, -22.3072) (-11.3588, -22.1386) knots 0 0 0 1 1 1
  spline S182 degree 2 poles (-11.3588, -22.1386) (-11.6258, -21.9746) (-11.9913, -21.6372) knots 0 0 0 1 1 1
  line L126 (-11.9913, -21.6372) -> (-12.8956, -20.7985)
  line L127 (-12.8956, -20.7985) -> (-12.8956, -22.3541)
  line L128 (-12.8956, -22.3541) -> (-13.2189, -22.3541)
  line L129 (-13.2189, -22.3541) -> (-13.2189, -20.0676)
  line L130 (-13.2189, -20.0676) -> (-11.832, -21.3514)
  spline S183 degree 2 poles (-11.832, -21.3514) (-11.4665, -21.6888) (-11.2557, -21.834) knots 0 0 0 1 1 1
  spline S184 degree 2 poles (-11.2557, -21.834) (-11.0448, -21.9793) (-10.7731, -21.9793) knots 0 0 0 1 1 1
  spline S185 degree 2 poles (-10.7731, -21.9793) (-10.5013, -21.9793) (-10.2952, -21.7637) knots 0 0 0 1 1 1
  spline S186 degree 2 poles (-10.2952, -21.7637) (-10.089, -21.5529) (-10.089, -21.2343) knots 0 0 0 1 1 1
  spline S187 degree 2 poles (-10.089, -21.2343) (-10.089, -20.9204) (-10.3046, -20.7095) knots 0 0 0 1 1 1
  spline S188 degree 2 poles (-10.3046, -20.7095) (-10.5154, -20.5034) (-10.909, -20.4706) knots 0 0 0 1 1 1
  line L131 (-16.8879, 23.6295) -> (-16.8879, 23.2132)
  line L132 (-16.8879, 23.2132) -> (-18.8865, 24.0801)
  line L133 (-18.8865, 24.0801) -> (-18.8865, 24.2018)
  line L134 (-18.8865, 24.2018) -> (-17.5178, 24.7847)
  line L135 (-17.5178, 24.7847) -> (-18.8865, 25.3569)
  line L136 (-18.8865, 25.3569) -> (-18.8865, 25.4829)
  line L137 (-18.8865, 25.4829) -> (-16.8879, 26.3584)
  line L138 (-16.8879, 26.3584) -> (-16.8879, 25.942)
  line L139 (-16.8879, 25.942) -> (-18.0794, 25.4274)
  line L140 (-18.0794, 25.4274) -> (-16.8879, 24.9278)
  line L141 (-16.8879, 24.9278) -> (-16.8879, 24.6395)
  line L142 (-16.8879, 24.6395) -> (-18.0794, 24.142)
  line L143 (-18.0794, 24.142) -> (-16.8879, 23.6295)
  line L144 (-16.8879, 20.4843) -> (-16.8879, 20.068)
  line L145 (-16.8879, 20.068) -> (-18.8865, 20.9349)
  line L146 (-18.8865, 20.9349) -> (-18.8865, 21.0566)
  line L147 (-18.8865, 21.0566) -> (-17.5178, 21.6395)
  line L148 (-17.5178, 21.6395) -> (-18.8865, 22.2117)
  line L149 (-18.8865, 22.2117) -> (-18.8865, 22.3377)
  line L150 (-18.8865, 22.3377) -> (-16.8879, 23.2132)
  line L151 (-16.8879, 23.2132) -> (-16.8879, 22.7968)
  line L152 (-16.8879, 22.7968) -> (-18.0794, 22.2822)
  line L153 (-18.0794, 22.2822) -> (-16.8879, 21.7826)
  line L154 (-16.8879, 21.7826) -> (-16.8879, 21.4943)
  line L155 (-16.8879, 21.4943) -> (-18.0794, 20.9968)
  line L156 (-18.0794, 20.9968) -> (-16.8879, 20.4843)
  line L157 (-16.8879, 17.3391) -> (-16.8879, 16.9228)
  line L158 (-16.8879, 16.9228) -> (-18.8865, 17.7897)
  line L159 (-18.8865, 17.7897) -> (-18.8865, 17.9114)
  line L160 (-18.8865, 17.9114) -> (-17.5178, 18.4943)
  line L161 (-17.5178, 18.4943) -> (-18.8865, 19.0666)
  line L162 (-18.8865, 19.0666) -> (-18.8865, 19.1925)
  line L163 (-18.8865, 19.1925) -> (-16.8879, 20.068)
  line L164 (-16.8879, 20.068) -> (-16.8879, 19.6516)
  line L165 (-16.8879, 19.6516) -> (-18.0794, 19.137)
  line L166 (-18.0794, 19.137) -> (-16.8879, 18.6374)
  line L167 (-16.8879, 18.6374) -> (-16.8879, 18.3491)
  line L168 (-16.8879, 18.3491) -> (-18.0794, 17.8516)
  line L169 (-18.0794, 17.8516) -> (-16.8879, 17.3391)
  spline S189 degree 2 poles (-18.3761, 16.4466) (-18.3761, 16.3377) (-18.4509, 16.2609) knots 0 0 0 1 1 1
  spline S190 degree 2 poles (-18.4509, 16.2609) (-18.5256, 16.184) (-18.6345, 16.184) knots 0 0 0 1 1 1
  spline S191 degree 2 poles (-18.6345, 16.184) (-18.7413, 16.184) (-18.8139, 16.2609) knots 0 0 0 1 1 1
  spline S192 degree 2 poles (-18.8139, 16.2609) (-18.8865, 16.3356) (-18.8865, 16.4466) knots 0 0 0 1 1 1
  spline S193 degree 2 poles (-18.8865, 16.4466) (-18.8865, 16.5555) (-18.8139, 16.6303) knots 0 0 0 1 1 1
  spline S194 degree 2 poles (-18.8139, 16.6303) (-18.7413, 16.705) (-18.6345, 16.705) knots 0 0 0 1 1 1
  spline S195 degree 2 poles (-18.6345, 16.705) (-18.5256, 16.705) (-18.4509, 16.6303) knots 0 0 0 1 1 1
  spline S196 degree 2 poles (-18.4509, 16.6303) (-18.3761, 16.5555) (-18.3761, 16.4466) knots 0 0 0 1 1 1
  line L170 (-17.426, 14.0786) -> (-18.8523, 14.0786)
  line L171 (-18.8523, 14.0786) -> (-18.8523, 14.4694)
  line L172 (-18.8523, 14.4694) -> (-17.7591, 14.4694)
  spline S197 degree 2 poles (-17.7591, 14.4694) (-17.4324, 14.4694) (-17.3043, 14.5569) knots 0 0 0 1 1 1
  spline S198 degree 2 poles (-17.3043, 14.5569) (-17.174, 14.6445) (-17.174, 14.8623) knots 0 0 0 1 1 1
  spline S199 degree 2 poles (-17.174, 14.8623) (-17.174, 14.984) (-17.2295, 15.0865) knots 0 0 0 1 1 1
  spline S200 degree 2 poles (-17.2295, 15.0865) (-17.285, 15.1868) (-17.426, 15.3171) knots 0 0 0 1 1 1
  line L173 (-17.426, 15.3171) -> (-18.8523, 15.3171)
  line L174 (-18.8523, 15.3171) -> (-18.8523, 15.7057)
  line L175 (-18.8523, 15.7057) -> (-16.8879, 15.7057)
  line L176 (-16.8879, 15.7057) -> (-16.8879, 15.3171)
  line L177 (-16.8879, 15.3171) -> (-17.1463, 15.3171)
  spline S201 degree 2 poles (-17.1463, 15.3171) (-16.8495, 15.0203) (-16.8495, 14.7363) knots 0 0 0 1 1 1
  spline S202 degree 2 poles (-16.8495, 14.7363) (-16.8495, 14.3626) (-17.2039, 14.1577) knots 0 0 0 1 1 1
  spline S203 degree 2 poles (-17.2039, 14.1577) (-16.8452, 13.8459) (-16.8452, 13.5064) knots 0 0 0 1 1 1
  spline S204 degree 2 poles (-16.8452, 13.5064) (-16.8452, 13.2203) (-17.0544, 13.0367) knots 0 0 0 1 1 1
  spline S205 degree 2 poles (-17.0544, 13.0367) (-17.2637, 12.8509) (-17.6929, 12.8509) knots 0 0 0 1 1 1
  line L178 (-17.6929, 12.8509) -> (-18.8523, 12.8509)
  line L179 (-18.8523, 12.8509) -> (-18.8523, 13.2395)
  line L180 (-18.8523, 13.2395) -> (-17.6886, 13.2395)
  spline S206 degree 2 poles (-17.6886, 13.2395) (-17.4431, 13.2395) (-17.3128, 13.3399) knots 0 0 0 1 1 1
  spline S207 degree 2 poles (-17.3128, 13.3399) (-17.1826, 13.4402) (-17.1826, 13.6281) knots 0 0 0 1 1 1
  spline S208 degree 2 poles (-17.1826, 13.6281) (-17.1826, 13.8694) (-17.426, 14.0786) knots 0 0 0 1 1 1
  spline S209 degree 2 poles (-16.0616, 12.1164) (-16.0616, 12.0203) (-16.1277, 11.952) knots 0 0 0 1 1 1
  spline S210 degree 2 poles (-16.1277, 11.952) (-16.1939, 11.8836) (-16.29, 11.8836) knots 0 0 0 1 1 1
  spline S211 degree 2 poles (-16.29, 11.8836) (-16.384, 11.8836) (-16.4523, 11.952) knots 0 0 0 1 1 1
  spline S212 degree 2 poles (-16.4523, 11.952) (-16.5206, 12.0203) (-16.5206, 12.1164) knots 0 0 0 1 1 1
  spline S213 degree 2 poles (-16.5206, 12.1164) (-16.5206, 12.2061) (-16.4523, 12.2744) knots 0 0 0 1 1 1
  spline S214 degree 2 poles (-16.4523, 12.2744) (-16.3818, 12.3427) (-16.29, 12.3427) knots 0 0 0 1 1 1
  spline S215 degree 2 poles (-16.29, 12.3427) (-16.2003, 12.3427) (-16.132, 12.2744) knots 0 0 0 1 1 1
  spline S216 degree 2 poles (-16.132, 12.2744) (-16.0616, 12.2061) (-16.0616, 12.1164) knots 0 0 0 1 1 1
  line L181 (-16.8879, 12.3085) -> (-16.8879, 11.9199)
  line L182 (-16.8879, 11.9199) -> (-18.8523, 11.9199)
  line L183 (-18.8523, 11.9199) -> (-18.8523, 12.3085)
  line L184 (-18.8523, 12.3085) -> (-16.8879, 12.3085)
  line L185 (-16.8879, 10.9698) -> (-17.1377, 10.9698)
  spline S217 degree 2 poles (-17.1377, 10.9698) (-16.8495, 10.7093) (-16.8495, 10.3783) knots 0 0 0 1 1 1
  spline S218 degree 2 poles (-16.8495, 10.3783) (-16.8495, 10.1947) (-16.9455, 10.0367) knots 0 0 0 1 1 1
  spline S219 degree 2 poles (-16.9455, 10.0367) (-17.0395, 9.8786) (-17.206, 9.7975) knots 0 0 0 1 1 1
  spline S220 degree 2 poles (-17.206, 9.7975) (-17.3705, 9.7142) (-17.7292, 9.7142) knots 0 0 0 1 1 1
  line L186 (-17.7292, 9.7142) -> (-18.8523, 9.7142)
  line L187 (-18.8523, 9.7142) -> (-18.8523, 10.1028)
  line L188 (-18.8523, 10.1028) -> (-17.7334, 10.1028)
  spline S221 degree 2 poles (-17.7334, 10.1028) (-17.4324, 10.1028) (-17.3043, 10.1947) knots 0 0 0 1 1 1
  spline S222 degree 2 poles (-17.3043, 10.1947) (-17.174, 10.2865) (-17.174, 10.5021) knots 0 0 0 1 1 1
  spline S223 degree 2 poles (-17.174, 10.5021) (-17.174, 10.7776) (-17.4495, 10.9698) knots 0 0 0 1 1 1
  line L189 (-17.4495, 10.9698) -> (-18.8523, 10.9698)
  line L190 (-18.8523, 10.9698) -> (-18.8523, 11.3669)
  line L191 (-18.8523, 11.3669) -> (-16.8879, 11.3669)
  line L192 (-16.8879, 11.3669) -> (-16.8879, 10.9698)
  spline S224 degree 2 poles (-16.0616, 8.9712) (-16.0616, 8.8751) (-16.1277, 8.8068) knots 0 0 0 1 1 1
  spline S225 degree 2 poles (-16.1277, 8.8068) (-16.1939, 8.7384) (-16.29, 8.7384) knots 0 0 0 1 1 1
  spline S226 degree 2 poles (-16.29, 8.7384) (-16.384, 8.7384) (-16.4523, 8.8068) knots 0 0 0 1 1 1
  spline S227 degree 2 poles (-16.4523, 8.8068) (-16.5206, 8.8751) (-16.5206, 8.9712) knots 0 0 0 1 1 1
  spline S228 degree 2 poles (-16.5206, 8.9712) (-16.5206, 9.0609) (-16.4523, 9.1292) knots 0 0 0 1 1 1
  spline S229 degree 2 poles (-16.4523, 9.1292) (-16.3818, 9.1975) (-16.29, 9.1975) knots 0 0 0 1 1 1
  spline S230 degree 2 poles (-16.29, 9.1975) (-16.2003, 9.1975) (-16.132, 9.1292) knots 0 0 0 1 1 1
  spline S231 degree 2 poles (-16.132, 9.1292) (-16.0616, 9.0609) (-16.0616, 8.9712) knots 0 0 0 1 1 1
  line L193 (-16.8879, 9.1633) -> (-16.8879, 8.7747)
  line L194 (-16.8879, 8.7747) -> (-18.8523, 8.7747)
  line L195 (-18.8523, 8.7747) -> (-18.8523, 9.1633)
  line L196 (-18.8523, 9.1633) -> (-16.8879, 9.1633)
  line L197 (-18.7114, 8.3093) -> (-18.2929, 8.3093)
  spline S232 degree 2 poles (-18.2929, 8.3093) (-18.4082, 8.1448) (-18.4808, 7.974) knots 0 0 0 1 1 1
  spline S233 degree 2 poles (-18.4808, 7.974) (-18.5512, 7.8011) (-18.5512, 7.6836) knots 0 0 0 1 1 1
  spline S234 degree 2 poles (-18.5512, 7.6836) (-18.5512, 7.5619) (-18.4915, 7.4744) knots 0 0 0 1 1 1
  spline S235 degree 2 poles (-18.4915, 7.4744) (-18.4317, 7.3868) (-18.3484, 7.3868) knots 0 0 0 1 1 1
  spline S236 degree 2 poles (-18.3484, 7.3868) (-18.263, 7.3868) (-18.2075, 7.4445) knots 0 0 0 1 1 1
  spline S237 degree 2 poles (-18.2075, 7.4445) (-18.1498, 7.5) (-18.0431, 7.6879) knots 0 0 0 1 1 1
  spline S238 degree 2 poles (-18.0431, 7.6879) (-17.8338, 8.0637) (-17.6865, 8.1811) knots 0 0 0 1 1 1
  spline S239 degree 2 poles (-17.6865, 8.1811) (-17.537, 8.2964) (-17.3619, 8.2964) knots 0 0 0 1 1 1
  spline S240 degree 2 poles (-17.3619, 8.2964) (-17.1356, 8.2964) (-16.9925, 8.1214) knots 0 0 0 1 1 1
  spline S241 degree 2 poles (-16.9925, 8.1214) (-16.8495, 7.9441) (-16.8495, 7.6665) knots 0 0 0 1 1 1
  spline S242 degree 2 poles (-16.8495, 7.6665) (-16.8495, 7.3783) (-17.0117, 7.0751) knots 0 0 0 1 1 1
  line L198 (-17.0117, 7.0751) -> (-17.3961, 7.0751)
  spline S243 degree 2 poles (-17.3961, 7.0751) (-17.1868, 7.421) (-17.1868, 7.6409) knots 0 0 0 1 1 1
  spline S244 degree 2 poles (-17.1868, 7.6409) (-17.1868, 7.7541) (-17.2359, 7.8246) knots 0 0 0 1 1 1
  spline S245 degree 2 poles (-17.2359, 7.8246) (-17.2829, 7.8929) (-17.3619, 7.8929) knots 0 0 0 1 1 1
  spline S246 degree 2 poles (-17.3619, 7.8929) (-17.4302, 7.8929) (-17.4922, 7.831) knots 0 0 0 1 1 1
  spline S247 degree 2 poles (-17.4922, 7.831) (-17.5541, 7.7669) (-17.6416, 7.6089) knots 0 0 0 1 1 1
  line L199 (-17.6416, 7.6089) -> (-17.7206, 7.4701)
  spline S248 degree 2 poles (-17.7206, 7.4701) (-17.9982, 6.979) (-18.3356, 6.979) knots 0 0 0 1 1 1
  spline S249 degree 2 poles (-18.3356, 6.979) (-18.5769, 6.979) (-18.7327, 7.169) knots 0 0 0 1 1 1
  spline S250 degree 2 poles (-18.7327, 7.169) (-18.8865, 7.3569) (-18.8865, 7.6537) knots 0 0 0 1 1 1
  spline S251 degree 2 poles (-18.8865, 7.6537) (-18.8865, 7.8288) (-18.8502, 7.9655) knots 0 0 0 1 1 1
  spline S252 degree 2 poles (-18.8502, 7.9655) (-18.8117, 8.1021) (-18.7114, 8.3093) knots 0 0 0 1 1 1
  line L200 (-19.8537, 6.5562) -> (-16.8879, 6.5562)
  line L201 (-16.8879, 6.5562) -> (-16.8879, 5.8751)
  spline S253 degree 2 poles (-16.8879, 5.8751) (-16.8879, 5.352) (-17.1484, 5.0616) knots 0 0 0 1 1 1
  spline S254 degree 2 poles (-17.1484, 5.0616) (-17.4089, 4.769) (-17.8765, 4.769) knots 0 0 0 1 1 1
  spline S255 degree 2 poles (-17.8765, 4.769) (-18.3185, 4.769) (-18.6025, 5.0445) knots 0 0 0 1 1 1
  spline S256 degree 2 poles (-18.6025, 5.0445) (-18.8865, 5.3178) (-18.8865, 5.7427) knots 0 0 0 1 1 1
  spline S257 degree 2 poles (-18.8865, 5.7427) (-18.8865, 5.9306) (-18.8032, 6.1591) knots 0 0 0 1 1 1
  line L202 (-18.8032, 6.1591) -> (-19.8537, 6.1591)
  line L203 (-19.8537, 6.1591) -> (-19.8537, 6.5562)
  line L204 (-17.2509, 5.8836) -> (-17.2509, 6.1591)
  line L205 (-17.2509, 6.1591) -> (-18.4594, 6.1591)
  spline S258 degree 2 poles (-18.4594, 6.1591) (-18.5512, 5.9797) (-18.5512, 5.7833) knots 0 0 0 1 1 1
  spline S259 degree 2 poles (-18.5512, 5.7833) (-18.5512, 5.51) (-18.3612, 5.337) knots 0 0 0 1 1 1
  spline S260 degree 2 poles (-18.3612, 5.337) (-18.1712, 5.1619) (-17.8722, 5.1619) knots 0 0 0 1 1 1
  spline S261 degree 2 poles (-17.8722, 5.1619) (-17.6801, 5.1619) (-17.5327, 5.2452) knots 0 0 0 1 1 1
  spline S262 degree 2 poles (-17.5327, 5.2452) (-17.3854, 5.3263) (-17.3192, 5.4694) knots 0 0 0 1 1 1
  spline S263 degree 2 poles (-17.3192, 5.4694) (-17.2509, 5.6103) (-17.2509, 5.8836) knots 0 0 0 1 1 1
  line L206 (-17.9043, 2.6701) -> (-17.9043, 4.0516)
  spline S264 degree 2 poles (-17.9043, 4.0516) (-18.1861, 4.0367) (-18.3527, 3.8637) knots 0 0 0 1 1 1
  spline S265 degree 2 poles (-18.3527, 3.8637) (-18.5192, 3.6886) (-18.5192, 3.4132) knots 0 0 0 1 1 1
  spline S266 degree 2 poles (-18.5192, 3.4132) (-18.5192, 3.0288) (-18.2801, 2.7043) knots 0 0 0 1 1 1
  line L207 (-18.2801, 2.7043) -> (-18.6601, 2.7043)
  spline S267 degree 2 poles (-18.6601, 2.7043) (-18.7797, 2.8836) (-18.831, 3.0609) knots 0 0 0 1 1 1
  spline S268 degree 2 poles (-18.831, 3.0609) (-18.8822, 3.2359) (-18.8822, 3.473) knots 0 0 0 1 1 1
  spline S269 degree 2 poles (-18.8822, 3.473) (-18.8822, 3.7975) (-18.7477, 3.9982) knots 0 0 0 1 1 1
  spline S270 degree 2 poles (-18.7477, 3.9982) (-18.6132, 4.1989) (-18.3868, 4.3206) knots 0 0 0 1 1 1
  spline S271 degree 2 poles (-18.3868, 4.3206) (-18.1584, 4.4402) (-17.8594, 4.4402) knots 0 0 0 1 1 1
  spline S272 degree 2 poles (-17.8594, 4.4402) (-17.411, 4.4402) (-17.1313, 4.1861) knots 0 0 0 1 1 1
  spline S273 degree 2 poles (-17.1313, 4.1861) (-16.8495, 3.932) (-16.8495, 3.5263) knots 0 0 0 1 1 1
  spline S274 degree 2 poles (-16.8495, 3.5263) (-16.8495, 3.1356) (-17.1228, 2.9028) knots 0 0 0 1 1 1
  spline S275 degree 2 poles (-17.1228, 2.9028) (-17.3961, 2.6701) (-17.8552, 2.6701) knots 0 0 0 1 1 1
  line L208 (-17.8552, 2.6701) -> (-17.9043, 2.6701)
  line L209 (-17.6715, 4.0431) -> (-17.6715, 3.0545)
  spline S276 degree 2 poles (-17.6715, 3.0545) (-17.4388, 3.0694) (-17.3128, 3.1932) knots 0 0 0 1 1 1
  spline S277 degree 2 poles (-17.3128, 3.1932) (-17.1868, 3.3171) (-17.1868, 3.5263) knots 0 0 0 1 1 1
  spline S278 degree 2 poles (-17.1868, 3.5263) (-17.1868, 3.7356) (-17.3128, 3.8701) knots 0 0 0 1 1 1
  spline S279 degree 2 poles (-17.3128, 3.8701) (-17.4388, 4.0025) (-17.6715, 4.0431) knots 0 0 0 1 1 1
  line L210 (-18.3932, 0.7762) -> (-18.7776, 0.7762)
  spline S280 degree 2 poles (-18.7776, 0.7762) (-18.8865, 1.0687) (-18.8865, 1.3484) knots 0 0 0 1 1 1
  spline S281 degree 2 poles (-18.8865, 1.3484) (-18.8865, 1.8096) (-18.6132, 2.0851) knots 0 0 0 1 1 1
  spline S282 degree 2 poles (-18.6132, 2.0851) (-18.3398, 2.3584) (-17.8808, 2.3584) knots 0 0 0 1 1 1
  spline S283 degree 2 poles (-17.8808, 2.3584) (-17.4174, 2.3584) (-17.1334, 2.0915) knots 0 0 0 1 1 1
  spline S284 degree 2 poles (-17.1334, 2.0915) (-16.8495, 1.8246) (-16.8495, 1.389) knots 0 0 0 1 1 1
  spline S285 degree 2 poles (-16.8495, 1.389) (-16.8495, 1.2374) (-16.8794, 1.1178) knots 0 0 0 1 1 1
  spline S286 degree 2 poles (-16.8794, 1.1178) (-16.9071, 0.9961) (-16.9861, 0.8189) knots 0 0 0 1 1 1
  line L211 (-16.9861, 0.8189) -> (-17.4003, 0.8189)
  spline S287 degree 2 poles (-17.4003, 0.8189) (-17.2124, 1.1135) (-17.2124, 1.3655) knots 0 0 0 1 1 1
  spline S288 degree 2 poles (-17.2124, 1.3655) (-17.2124, 1.6281) (-17.3982, 1.7968) knots 0 0 0 1 1 1
  spline S289 degree 2 poles (-17.3982, 1.7968) (-17.5818, 1.9655) (-17.868, 1.9655) knots 0 0 0 1 1 1
  spline S290 degree 2 poles (-17.868, 1.9655) (-18.169, 1.9655) (-18.3463, 1.784) knots 0 0 0 1 1 1
  spline S291 degree 2 poles (-18.3463, 1.784) (-18.5235, 1.6004) (-18.5235, 1.2908) knots 0 0 0 1 1 1
  spline S292 degree 2 poles (-18.5235, 1.2908) (-18.5235, 1.0666) (-18.3932, 0.7762) knots 0 0 0 1 1 1
  line L212 (-17.1996, 0.6096) -> (-16.4822, -0.1206)
  line L213 (-16.4822, -0.1206) -> (-16.8879, -0.1206)
  line L214 (-16.8879, -0.1206) -> (-16.8879, -0.742)
  line L215 (-16.8879, -0.742) -> (-17.2381, -0.742)
  line L216 (-17.2381, -0.742) -> (-17.2381, -0.1206)
  line L217 (-17.2381, -0.1206) -> (-18.2011, -0.1206)
  spline S293 degree 2 poles (-18.2011, -0.1206) (-18.5384, -0.1206) (-18.5384, -0.4004) knots 0 0 0 1 1 1
  spline S294 degree 2 poles (-18.5384, -0.4004) (-18.5384, -0.6096) (-18.3975, -0.8423) knots 0 0 0 1 1 1
  line L218 (-18.3975, -0.8423) -> (-18.7605, -0.8423)
  spline S295 degree 2 poles (-18.7605, -0.8423) (-18.8865, -0.6181) (-18.8865, -0.3534) knots 0 0 0 1 1 1
  spline S296 degree 2 poles (-18.8865, -0.3534) (-18.8865, -0.0865) (-18.7306, 0.0907) knots 0 0 0 1 1 1
  spline S297 degree 2 poles (-18.7306, 0.0907) (-18.6836, 0.1463) (-18.626, 0.1826) knots 0 0 0 1 1 1
  spline S298 degree 2 poles (-18.626, 0.1826) (-18.5662, 0.2189) (-18.4722, 0.2445) knots 0 0 0 1 1 1
  spline S299 degree 2 poles (-18.4722, 0.2445) (-18.3761, 0.268) (-18.1092, 0.268) knots 0 0 0 1 1 1
  line L219 (-18.1092, 0.268) -> (-17.2381, 0.268)
  line L220 (-17.2381, 0.268) -> (-17.2381, 0.6096)
  line L221 (-17.2381, 0.6096) -> (-17.1996, 0.6096)
  line L222 (-16.8879, -1.5384) -> (-17.3384, -1.5384)
  line L223 (-17.3384, -1.5384) -> (-17.3043, -1.5598)
  spline S300 degree 2 poles (-17.3043, -1.5598) (-16.8495, -1.8416) (-16.8495, -2.1235) knots 0 0 0 1 1 1
  spline S301 degree 2 poles (-16.8495, -2.1235) (-16.8495, -2.3434) (-17.0715, -2.5826) knots 0 0 0 1 1 1
  line L224 (-17.0715, -2.5826) -> (-17.4132, -2.3776)
  spline S302 degree 2 poles (-17.4132, -2.3776) (-17.221, -2.1747) (-17.221, -2.0018) knots 0 0 0 1 1 1
  spline S303 degree 2 poles (-17.221, -2.0018) (-17.221, -1.8139) (-17.4003, -1.6751) knots 0 0 0 1 1 1
  spline S304 degree 2 poles (-17.4003, -1.6751) (-17.5797, -1.5384) (-17.8253, -1.5384) knots 0 0 0 1 1 1
  line L225 (-17.8253, -1.5384) -> (-18.8523, -1.5384)
  line L226 (-18.8523, -1.5384) -> (-18.8523, -1.1477)